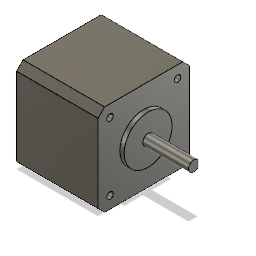
EggBot (Autodesk Fusion 360 archive; units mm, degrees)
design "Nema17"
Autodesk Fusion 360 part; units mm, degrees
sketch "Skizze1" plane through (0, 0, 0) normal (1, 0, 0) x (0, 0, -1)
  line L0 (21, 21) -> (-21, 21)
  line L1 (-21, 21) -> (-21, -21)
  line L2 (-21, -21) -> (21, -21)
  line L3 (21, -21) -> (21, 21)
  line L4 (21, 21) -> (-21, -21) construction
  line L5 (-21, 21) -> (21, -21) construction
  line L6 (15.5, -15.5) -> (-15.5, -15.5)
  line L7 (-15.5, -15.5) -> (-15.5, 15.5)
  line L8 (-15.5, 15.5) -> (15.5, 15.5)
  line L9 (15.5, 15.5) -> (15.5, -15.5)
  line L10 (15.5, -15.5) -> (-15.5, 15.5) construction
  line L11 (-15.5, -15.5) -> (15.5, 15.5) construction
  circle A0 centre (15.5, -15.5) radius 1.5
  circle A1 centre (-15.5, -15.5) radius 1.5
  circle A2 centre (-15.5, 15.5) radius 1.5
  circle A3 centre (15.5, 15.5) radius 1.5
  circle A4 centre (0, 0) radius 11
  circle A5 centre (0, 0) radius 2.5
  line L12 (0, 0) -> (2, 0)
  line L13 (2, 0) -> (2, 1.5)
  line L14 (2, 0) -> (2, -1.5)
  dimension "d1" = 42
  dimension "d2" = 42
  dimension "d5" = 31
  dimension "d6" = 31
  dimension "d7" = 3
  dimension "d8" = 3
  dimension "d9" = 3
  dimension "d10" = 3
  dimension "d13" = 22
  dimension "d16" = 5
  dimension "d20" = 2
  constraint perpendicular L0 L1
  constraint parallel L0 L2
  constraint parallel L1 L3
  constraint horizontal L0
  constraint coincident L4 A4.centre
  constraint coincident L5 A4.centre
  constraint coincident A4.centre A5.centre
  constraint perpendicular L6 L7
  constraint parallel L6 L8
  constraint parallel L7 L9
  constraint horizontal L6
  constraint coincident L10 A4.centre
  constraint coincident L11 A4.centre
  constraint coincident L6.start L9.end
  constraint coincident L6.end L7.start
  constraint coincident L7.end L8.start
  constraint coincident L8.end L9.start
  constraint concentric A4 A5
  constraint horizontal L12
  constraint coincident A5 L13.end
  constraint perpendicular L12 L13
  constraint coincident A5 L14.end
  constraint perpendicular L12 L14
  measures "d1" distance of L0.end L1.end
  measures "d2" distance of L1.end L2.end
  measures "d5" distance of L6.end L7.end
  measures "d6" distance of L7.end L8.end
  measures "d7" diameter of A0
  measures "d8" diameter of A1
  measures "d9" diameter of A2
  measures "d10" diameter of A3
  measures "d13" diameter of A4
  measures "d16" diameter of A5
  measures "d20" distance of A4.centre L12.end
extrude "Extrusion1" add sketch "Skizze1" against normal blind 37.5 contours L0 L1 L2 L3 | L6 L7 A1 | L6 L7 L8 L9 A0 A1 A2 A3 | L6 L7 A1 | L6 L9 A0 | L6 L9 A0 | L7 L8 A2 | L7 L8 A2 | L8 L9 A3 | L8 L9 A3 | A4 | A5 L13 L14 | A5 L13 L14
extrude "Extrusion2" cut sketch "Skizze1" against normal blind 4 contours L6 L7 A1 | L6 L7 A1 | L6 L9 A0 | L6 L9 A0 | L7 L8 A2 | L7 L8 A2 | L8 L9 A3 | L8 L9 A3
extrude "Extrusion3" add sketch "Skizze1" along normal blind 2 contours A4 | A5 L13 L14 | A5 L13 L14
extrude "Extrusion4" add sketch "Skizze1" along normal blind 23 contours A5 L13 L14 picked at (-0.991, 0.122)
chamfer "Fase1" distance 3 angle 45 4 edges at (-18.75, 21, 21) (-18.75, 21, -21) (-18.75, -21, -21) (-18.75, -21, 21)

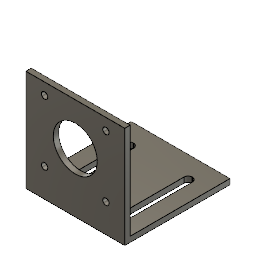
design "motor mount"
Autodesk Fusion 360 part; units mm, degrees
sketch "Skizze1" plane through (0, 0, 0) normal (0, 1, 0) x (1, 0, 0)
  line L0 (15.5, 11.2) -> (-15.5, 11.2)
  line L1 (-15.5, 11.2) -> (-15.5, -19.8)
  line L2 (-15.5, -19.8) -> (15.5, -19.8)
  line L3 (15.5, -19.8) -> (15.5, 11.2)
  line L4 (15.5, 11.2) -> (-15.5, -19.8) construction
  line L5 (-15.5, 11.2) -> (15.5, -19.8) construction
  line L6 (25, 25.7) -> (-25, 25.7)
  line L7 (-25, 25.7) -> (-25, -25.7)
  line L8 (-25, -25.7) -> (25, -25.7)
  line L9 (25, -25.7) -> (25, 25.7)
  line L10 (25, 25.7) -> (-25, -25.7) construction
  line L11 (-25, 25.7) -> (25, -25.7) construction
  circle A0 centre (0, -4.3) radius 11.1
  circle A1 centre (-15.5, 11.2) radius 1.6
  circle A2 centre (15.5, 11.2) radius 1.6
  circle A3 centre (-15.5, -19.8) radius 1.6
  circle A4 centre (15.5, -19.8) radius 1.6
  line L12 (0, -19.8) -> (0, -25.7)
  line L13 (25, 25.7) -> (-25, 25.7)
  line L14 (-25, 25.7) -> (-25, 76.2)
  line L15 (-25, 76.2) -> (25, 76.2)
  line L16 (25, 76.2) -> (25, 25.7)
  line L17 (25, 76.2) -> (25, 67.2)
  line L18 (25, 67.2) -> (-25, 67.2)
  line L19 (25, 67.2) -> (17, 67.2)
  line L20 (-25, 67.2) -> (-17, 67.2)
  line L21 (-15, 67.2) -> (-14.7, 67.2)
  line L22 (-12.7, 65.2) -> (-12.7, 35.2)
  line L23 (-14.7, 33.2) -> (-15, 33.2)
  line L24 (-17, 35.2) -> (-17, 65.2)
  line L25 (15, 67.2) -> (14.7, 67.2)
  line L26 (12.7, 65.2) -> (12.7, 35.2)
  line L27 (14.7, 33.2) -> (15, 33.2)
  line L28 (17, 35.2) -> (17, 65.2)
  arc A5 (-15, 67.2) -> (-17, 65.2) centre (-15, 65.2) ccw
  arc A6 (-12.7, 65.2) -> (-14.7, 67.2) centre (-14.7, 65.2) ccw
  arc A7 (-17, 35.2) -> (-15, 33.2) centre (-15, 35.2) ccw
  arc A8 (-14.7, 33.2) -> (-12.7, 35.2) centre (-14.7, 35.2) ccw
  arc A9 (12.7, 35.2) -> (14.7, 33.2) centre (14.7, 35.2) ccw
  arc A10 (15, 33.2) -> (17, 35.2) centre (15, 35.2) ccw
  arc A11 (14.7, 67.2) -> (12.7, 65.2) centre (14.7, 65.2) ccw
  arc A12 (17, 65.2) -> (15, 67.2) centre (15, 65.2) ccw
  point P0 (0, -4.3)
  point P1 (-12.7, 67.2)
  point P2 (-17, 33.2)
  point P3 (12.7, 67.2)
  point P4 (17, 33.2)
  dimension "d1" = 31
  dimension "d2" = 31
  dimension "d3" = 50
  dimension "d4" = 51.4
  dimension "d5" = 22.2
  dimension "d6" = 3.2
  dimension "d7" = 3.2
  dimension "d8" = 3.2
  dimension "d9" = 3.2
  dimension "d11" = 5.9
  dimension "d12" = 50.5
  dimension "d13" = 9
  dimension "d14" = 8
  dimension "d15" = 8
  dimension "d16" = 4.3
  dimension "d17" = 34
  dimension "d18" = 34
  dimension "d19" = 4.3
  dimension "d20" = 2
  dimension "d21" = 2
  dimension "d22" = 2
  dimension "d23" = 2
  dimension "d24" = 2
  dimension "d25" = 2
  dimension "d26" = 2
  dimension "d27" = 2
  constraint perpendicular L0 L1
  constraint parallel L0 L2
  constraint parallel L1 L3
  constraint horizontal L0
  constraint perpendicular L6 L7
  constraint parallel L6 L8
  constraint parallel L7 L9
  constraint horizontal L6
  constraint coincident L10 origin
  constraint coincident L11 origin
  constraint coincident L0.end L1.start
  constraint coincident L0.start L3.end
  constraint coincident L1.end L2.start
  constraint coincident L2.end L3.start
  constraint midpoint L2 L12.start
  constraint midpoint L8 L12.end
  constraint midpoint L4 P0
  constraint coincident P0 A0.centre
  constraint perpendicular L8 L12
  constraint horizontal L13
  constraint vertical L14
  constraint horizontal L15
  constraint vertical L16
  constraint perpendicular L15 L17
  constraint coincident L14 L18.end
  constraint perpendicular L14 L18
  constraint perpendicular L16 L19
  constraint perpendicular L14 L20
  constraint horizontal L21
  constraint vertical L22
  constraint horizontal L23
  constraint vertical L24
  constraint horizontal L25
  constraint vertical L26
  constraint horizontal L27
  constraint vertical L28
  constraint coincident L20.end L24
  constraint coincident L20.end L21
  constraint tangent L24 A5
  constraint tangent L21 A5
  constraint coincident P1 L22
  constraint coincident P1 L21
  constraint tangent L22 A6
  constraint tangent L21 A6
  constraint coincident P2 L24
  constraint coincident P2 L23
  constraint tangent L24 A7
  constraint tangent L23 A7
  constraint tangent L22 A8
  constraint tangent L23 A8
  constraint tangent L26 A9
  constraint tangent L27 A9
  constraint coincident P4 L28
  constraint coincident P4 L27
  constraint tangent L28 A10
  constraint tangent L27 A10
  constraint coincident P3 L26
  constraint coincident P3 L25
  constraint tangent L26 A11
  constraint tangent L25 A11
  constraint coincident L19.end L28
  constraint coincident L19.end L25
  constraint tangent L28 A12
  constraint tangent L25 A12
  measures "d1" distance of L1.end L2.end
  measures "d2" distance of L0.end L1.end
  measures "d3" distance of L7.end L8.end
  measures "d4" distance of L6.end L7.end
  measures "d5" diameter of A0
  measures "d6" diameter of A1
  measures "d7" diameter of A2
  measures "d8" diameter of A3
  measures "d9" diameter of A4
  measures "d11" distance of L12.start L12.end
  measures "d12" distance of L6.start L15.end
  measures "d13" distance of L15.end L17.end
  measures "d14" distance of L17.end L19.end
  measures "d15" distance of L18.end L20.end
  measures "d16" distance of L20.end P1
  measures "d17" distance of L20.end P2
  measures "d18" distance of L19.end P4
  measures "d19" distance of L19.end P3
  measures "d20" radius of A5
  measures "d21" radius of A6
  measures "d22" radius of A7
  measures "d23" radius of A8
  measures "d24" radius of A9
  measures "d25" radius of A10
  measures "d26" radius of A11
  measures "d27" radius of A12
extrude "Extrusion1" add sketch "Skizze1" against normal blind 2.8 contours L6 L13 L14 L16 L18 L19 L20 L22 L23 L24 L26 L27 L28 A5 A6 A7 A8 A9 A10 A11 A12 | L14 L15 L16 L17 L18 L19 L20 L21 L25 makes body 1
extrude "Extrusion2" add sketch "Skizze1" against normal blind 2.8 separate body contours L0 L1 L2 L3 A1 A2 A3 A4 | L6 L7 L8 L9 L13 makes body 2
move_body "Verschieben1" bodies 2 to x (1, 0, 0) y (0, 0, -1) z (0, 1, 0) at (0, 22.9, -28.5)
move_body "Verschieben2" bodies 2 to x (1, 0, 0) y (0, 1, 0) z (0, 0, 1) at (0, 0, 2.8)
combine "Kombinieren1" operation add target body 1 tool bodies 2
face "Fläche1" [suppressed]
other "Biegung1"
named bodies: "motor mount"
